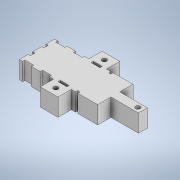
# Autodesk Inventor part: v8_Burrow_Base_Detachable_EXT_LICK_SPOUT
Saved by Autodesk Inventor 2020.4 (Build 244396010, 396A)
## iProperties
Created: 2021-09-30
Part Number: v8_Burrow_Base_Detachable_EXT_LICK_SPOUT
Material: Generic
Document SubType Name: Sheet Metal
Designer: YUSTE
Density: 1 g/cm^3
Sheet Metal Rule: Default
Appearance: Default
Author: YUSTE
Autodesk Inventor part; units mm, degrees
ref_plane "YZ Plane" through (0, 0, 0) normal (1, 0, 0) x (0, 1, 0)
ref_plane "XZ Plane" through (0, 0, 0) normal (0, 1, 0) x (-1, 0, 0)
ref_plane "XY Plane" through (0, 0, 0) normal (0, 0, 1) x (1, 0, 0)
sketch "Sketch1" plane through (0, 0, 0) normal (0, 1, 0) x (-1, 0, 0)
  line L0 (0, 0) -> (101.6, 0)
  line L1 (101.6, 0) -> (101.6, 50.8)
  line L2 (101.6, 50.8) -> (0, 50.8)
  line L3 (0, 50.8) -> (0, 0)
  line L4 (101.6, 0) -> (20.6375, 0)
  line L5 (20.6375, 50.8) -> (101.6, 50.8)
  line L6 (101.6, 50.8) -> (101.6, 0)
  line L7 (20.6375, 0) -> (0, 0)
  line L8 (0, 0) -> (0, 12.7)
  line L9 (0, 12.7) -> (20.6375, 12.7)
  line L10 (20.6375, 12.7) -> (20.6375, 0)
  line L11 (20.6375, 50.8) -> (0, 50.8)
  line L12 (0, 50.8) -> (0, 38.1)
  line L13 (0, 38.1) -> (20.6375, 38.1)
  line L14 (20.6375, 38.1) -> (20.6375, 50.8)
  line L15 (96.8375, 0) -> (84.1375, 0)
  line L16 (84.1375, 0) -> (84.1375, 3.175)
  line L17 (84.1375, 3.175) -> (96.8375, 3.175)
  line L18 (96.8375, 3.175) -> (96.8375, 0)
  line L19 (71.4375, 0) -> (58.7375, 0)
  line L20 (58.7375, 0) -> (58.7375, 3.175)
  line L21 (58.7375, 3.175) -> (71.4375, 3.175)
  line L22 (71.4375, 3.175) -> (71.4375, 0)
  line L23 (46.0375, 0) -> (33.3375, 0)
  line L24 (33.3375, 0) -> (33.3375, 3.175)
  line L25 (33.3375, 3.175) -> (46.0375, 3.175)
  line L26 (46.0375, 3.175) -> (46.0375, 0)
  line L27 (96.8375, 50.8) -> (84.1375, 50.8)
  line L28 (84.1375, 50.8) -> (84.1375, 47.625)
  line L29 (84.1375, 47.625) -> (96.8375, 47.625)
  line L30 (96.8375, 47.625) -> (96.8375, 50.8)
  line L31 (71.4375, 50.8) -> (58.7375, 50.8)
  line L32 (58.7375, 50.8) -> (58.7375, 47.625)
  line L33 (58.7375, 47.625) -> (71.4375, 47.625)
  line L34 (71.4375, 47.625) -> (71.4375, 50.8)
  line L35 (101.6, 38.1) -> (98.425, 38.1)
  line L36 (98.425, 38.1) -> (98.425, 31.75)
  line L37 (98.425, 31.75) -> (101.6, 31.75)
  line L38 (101.6, 31.75) -> (101.6, 38.1)
  line L39 (101.6, 19.05) -> (98.425, 19.05)
  line L40 (98.425, 19.05) -> (98.425, 12.7)
  line L41 (98.425, 12.7) -> (101.6, 12.7)
  line L42 (101.6, 12.7) -> (101.6, 19.05)
  line L43 (46.0375, 50.8) -> (46.0375, 47.625)
  line L44 (46.0375, 47.625) -> (33.3375, 47.625)
  line L45 (33.3375, 47.625) -> (33.3375, 50.8)
  line L46 (33.3375, 50.8) -> (46.0375, 50.8)
  line L47 (26.9875, 0) -> (52.3875, 0)
  line L48 (52.3875, 0) -> (52.3875, -19.05)
  line L49 (52.3875, -19.05) -> (26.9875, -19.05)
  line L50 (26.9875, -19.05) -> (26.9875, 0)
  line L51 (26.9875, 50.8) -> (26.9875, 69.85)
  line L52 (26.9875, 69.85) -> (52.3875, 69.85)
  line L53 (52.3875, 69.85) -> (52.3875, 50.8)
  line L54 (52.3875, 50.8) -> (26.9875, 50.8)
  circle A0 centre (39.6875, -9.525) radius 3.302
  circle A1 centre (39.6875, 60.325) radius 3.302
  line L55 (0, 19.05) -> (0, 31.75)
  line L56 (0, 31.75) -> (-50.8, 31.75)
  line L57 (-50.8, 31.75) -> (-50.8, 19.05)
  line L58 (-50.8, 19.05) -> (0, 19.05)
  circle A2 centre (-43.5387, 25.4) radius 3.302
  line L59 (26.9875, 50.8) -> (24.8905, 50.8)
  line L60 (26.9875, 0) -> (25.4, 0)
  line L61 (20.6375, 0) -> (17.4625, 0)
  line L62 (17.4625, 0) -> (17.4625, 3.175)
  line L63 (17.4625, 3.175) -> (20.6375, 3.175)
  line L64 (20.6375, 3.175) -> (20.6375, 0)
  line L65 (20.6375, 50.8) -> (17.4625, 50.8)
  line L66 (17.4625, 50.8) -> (17.4625, 47.625)
  line L67 (17.4625, 47.625) -> (20.6375, 47.625)
  line L68 (20.6375, 47.625) -> (20.6375, 50.8)
  line L69 (20.6375, 0) -> (-11.1125, 0)
  line L70 (-11.1125, 0) -> (-11.1125, 50.8)
  line L71 (-11.1125, 50.8) -> (20.6375, 50.8)
  line L72 (20.6375, 50.8) -> (20.6375, 0)
  point P0 (96.8375, 0)
  point P1 (96.8375, 50.8)
  point P2 (84.1375, 50.8)
  point P3 (71.4375, 50.8)
  point P4 (58.7375, 50.8)
  point P5 (46.0375, 50.8)
  point P6 (33.3375, 50.8)
  point P7 (33.3375, 0)
  point P8 (46.0375, 0)
  point P9 (58.7375, 0)
  point P10 (71.4375, 0)
  point P11 (84.1375, 0)
  point P12 (26.9875, 0)
  point P13 (52.3875, 0)
  point P14 (52.3875, 50.8)
  point P15 (26.9875, 50.8)
  point P16 (17.4625, 0)
  point P17 (0, 50.8)
  point P18 (-11.1125, 31.75)
  point P19 (-11.1125, 19.05)
  dimension "d56" = 101.6
  dimension "d57" = 50.8
  dimension "d59" = 50.8
  dimension "d60" = 12.7
  dimension "d61" = 12.7
  dimension "d62" = 12.7
  dimension "d63" = 3.175
  dimension "d64" = 12.7
  dimension "d65" = 3.175
  dimension "d66" = 12.7
  dimension "d67" = 4.7625
  dimension "d68" = 12.7
  dimension "d69" = 3.175
  dimension "d70" = 12.7
  dimension "d71" = 12.7
  dimension "d72" = 3.175
  dimension "d73" = 12.7
  dimension "d74" = 3.175
  dimension "d77" = 4.7625
  dimension "d78" = 12.7
  dimension "d79" = 3.175
  dimension "d80" = 6.35
  dimension "d81" = 12.7
  dimension "d82" = 3.175
  dimension "d83" = 6.35
  dimension "d84" = 12.7
  dimension "d86" = 44.45
  dimension "d89" = 3.175
  dimension "d90" = 12.7
  dimension "d91" = 12.7
  dimension "d94" = 25.4
  dimension "d99" = 25.4
  dimension "d116" = 6.604
  dimension "d117" = 9.525
  dimension "d118" = 6.604
  dimension "d119" = 9.525
  dimension "d122" = 9.525
  dimension "d123" = 9.525
  dimension "d128" = 12.7
  dimension "d129" = 50.8
  dimension "d130" = 6.604
  dimension "d131" = 6.35
  dimension "d132" = 12.7
  dimension "d134" = 12.7
  dimension "d141" = 25.4
  dimension "d144" = 6.35
  dimension "d145" = 6.35
  dimension "d147" = 3.175
  dimension "d148" = 3.175
  dimension "d149" = 3.175
  dimension "d150" = 3.175
  dimension "d151" = 12.7
  dimension "d152" = 12.7
  dimension "d155" = 31.75
  constraints: 144 end point, 34 parallel, 22 perpendicular, 15 point on line, 3 centre point, 3 horizontal, 11 other
  measures "d56" distance of L0.start L0.end
  measures "d57" distance of L1.end L0.end
  measures "d59" distance of L7.start L5.start
  measures "d60" distance of L0.start L8.end
  measures "d61" distance of L12.end L2.end
  measures "d62" distance of L15.start L15.end
  measures "d63" distance of L15.end L16.end
  measures "d64" distance of L19.start L19.end
  measures "d65" distance of L19.end L20.end
  measures "d66" distance between parallel lines of L16 L22
  measures "d67" distance between parallel lines of L1 L18
  measures "d68" distance of L23.start L23.end
  measures "d69" distance of L23.end L24.end
  measures "d70" distance between parallel lines of L26 L20
  measures "d71" distance of L27.start L27.end
  measures "d72" distance of L28.end L27.end
  measures "d73" distance of L31.start L31.end
  measures "d74" distance of L32.end L31.end
  measures "d77" distance between parallel lines of L1 L30
  measures "d78" distance between parallel lines of L34 L28
  measures "d79" distance of L35.start L35.end
  measures "d80" distance of L36.end L35.end
  measures "d81" distance between parallel lines of L2 L35
  measures "d82" distance of L39.start L39.end
  measures "d83" distance of L40.end L39.end
  measures "d84" distance between parallel lines of L0 L41
  measures "d86" distance between parallel lines of L29 L17
  measures "d89" distance of L43.start L43.end
  measures "d90" distance of L43.end L44.end
  measures "d91" distance between parallel lines of L43 L32
  measures "d94" distance of L47.start L47.end
  measures "d99" distance of L51.end L52.end
  measures "d116" diameter of A0
  measures "d117" distance from line of L19 A0.centre
  measures "d118" diameter of A1
  measures "d119" distance from line of L31 A1.centre
  measures "d122" distance from line of L49 A0.centre
  measures "d123" distance from line of L52 A1.centre
  measures "d128" distance of L55.start L55.end
  measures "d129" distance of L56.end L55.end
  measures "d130" diameter of A2
  measures "d131" distance from line of L58 A2.centre
  measures "d132" distance from line of L50 A0.centre
  measures "d134" distance from line of L51 A1.centre
  measures "d141" distance from line of L11 A2.centre
  measures "d144" distance between parallel lines of L26 L48
  measures "d145" distance between parallel lines of L43 L53
  measures "d147" distance of L7.start L61.end
  measures "d148" distance of L61.end L62.end
  measures "d149" distance of L5.start L65.end
  measures "d150" distance of L66.end L65.end
  measures "d151" distance between parallel lines of L24 L10
  measures "d152" distance between parallel lines of L14 L45
  measures "d155" distance of L7.start L69.end
extrude "Extrusion10" add sketch "Sketch1" along normal blind 25.4 contours L3 L9 L10 L63 L62 L0 | L69 L70 L58 L3 | L3 L13 L72 L9 | L10 L72 L14 L2 L45 L44 L43 L32 L33 L34 L28 L29 L30 L1 L35 L36 L37 L39 L40 L41 L0 L18 L17 L16 L22 L21 L20 L26 L25 L24 | L58 L70 L56 L3 | L58 L57 L56 L70 | L56 L70 L71 L3 | L13 L3 L2 L66 L67 L14 | L0 L48 L49 L50 | L51 L52 L53 L2
equation "\"BendRadius\" = Thickness"
equation "\"BendReliefWidth\" = Thickness"
equation "\"BendReliefDepth\" = 0.5 * Thickness"
equation "\"CornerReliefSize\" = 4 * Thickness"
equation "\"MinimumRemnant\" = 2 * Thickness"
equation "\"TransitionRadius\" = BendRadius"
equation "\"JacobiRadiusSize\" = BendRadius"
equation "\"GapSize\" = Thickness"
equation "\"Thickness\" = 3.048"
body "Solid14"
